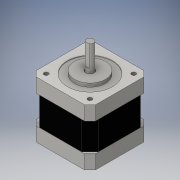
# Autodesk Inventor part: nema17_40mm
Saved by Autodesk Inventor 2016 (Build 200138000, 138)
## iProperties
Created: 2016-06-20
Part Number: nema17_40mm
Material: Generic
Document SubType Name: Modeling
Designer: brent
Density: 1 g/cm^3
Appearance: Aluminum - Dark
Author: brent
Autodesk Inventor part; units mm, degrees
ref_plane "YZ Plane" through (0, 0, 0) normal (1, 0, 0) x (0, 1, 0)
ref_plane "XZ Plane" through (0, 0, 0) normal (0, 1, 0) x (-1, 0, 0)
sketch "Sketch1" plane through (0, 0, 0) normal (0, 1, 0) x (-1, 0, 0)
  line L0 (-21, 21) -> (21, 21)
  line L1 (21, 21) -> (21, -21)
  line L2 (21, -21) -> (-21, -21)
  line L3 (-21, -21) -> (-21, 21)
  line L4 (-21, 21) -> (21, -21) construction
  line L5 (21, 21) -> (-21, -21) construction
  point P0 (0, 0)
  dimension "d0" = 42
  dimension "d1" = 42
  constraints: 12 end point, 2 midpoint, 2 parallel, 1 horizontal, 1 perpendicular
  measures "d0" distance of L1.end L2.end
  measures "d1" distance of L0.end L1.end
extrude "Extrusion1" add sketch "Sketch1" along normal blind 40
ref_plane "Work Plane1" through (0, 20, 0) normal (0, 1, 0) x (1, 0, 0)
sketch "Sketch2" plane through (0, 40, 0) normal (0, 1, 0) x (1, 0, 0)
  line L0 (0, -38.0423) -> (-38.0423, 0)
  line L1 (-38.0423, 0) -> (0, 38.0423)
  line L2 (0, 38.0423) -> (38.0423, 0)
  line L3 (38.0423, 0) -> (0, -38.0423)
  line L4 (0, -38.0423) -> (0, 38.0423) construction
  line L5 (-38.0423, 0) -> (38.0423, 0) construction
  line L6 (-21, 21) -> (-21, -21) projected
  circle A0 centre (0, 0) radius 250
  dimension "d4" = 53.8
  dimension "d5" = 53.8
  dimension "d6" = 500
  constraints: 12 end point, 2 midpoint, 2 parallel, 2 perpendicular, 1 centre point, 1 coincident
  measures "d4" distance of L0.end L1.end
  measures "d5" distance of L1.end L2.end
  measures "d6" diameter of A0
extrude "Extrusion2" cut sketch "Sketch2" against normal blind 10
sketch "Sketch3" plane through (0, 20, 0) normal (0, 1, 0) x (1, 0, 0)
  line L0 (-20.9, -20.9) -> (20.9, -20.9)
  line L1 (20.9, -20.9) -> (20.9, 20.9)
  line L2 (20.9, 20.9) -> (-20.9, 20.9)
  line L3 (-20.9, 20.9) -> (-20.9, -20.9)
  line L4 (-21, -21) -> (-21, -17.0423) projected
  line L5 (21, -21) -> (17.0423, -21) projected
  line L6 (21, 21) -> (21, 17.0423) projected
  line L7 (-21, 21) -> (-17.0423, 21) projected
  circle A0 centre (0, 0) radius 200
  dimension "d9" = 0.1
  dimension "d10" = 0.1
  dimension "d11" = 0.1
  dimension "d12" = 0.1
  dimension "d13" = 400
  constraints: 8 end point, 2 parallel, 1 centre point, 1 coincident, 1 horizontal, 1 perpendicular
  measures "d9" distance between parallel lines of L4 L3
  measures "d10" distance between parallel lines of L5 L0
  measures "d11" distance between parallel lines of L6 L1
  measures "d12" distance between parallel lines of L7 L2
  measures "d13" diameter of A0
extrude "Extrusion3" cut sketch "Sketch3" along normal up to surface (10 mm away)
chamfer "Chamfer1" distance 6 angle 45 4 edges at (20.9, 25, 20.9) (20.9, 25, -20.9) (-20.9, 25, 20.9) (-20.9, 25, -20.9)
mirror "Mirror1" about plane through (0, 20, 0) normal (0, 1, 0) of "Extrusion3", "Extrusion2", "Chamfer1"
sketch "Sketch4" plane through (0, 40, 0) normal (0, 1, 0) x (1, 0, 0)
  circle A0 centre (0, 0) radius 11
  dimension "d19" = 22
  constraints: 1 centre point, 1 coincident
  measures "d19" diameter of A0
extrude "Extrusion4" add sketch "Sketch4" along normal blind 2
sketch "Sketch5" plane through (0, 40, 0) normal (0, 1, 0) x (1, 0, 0)
  circle A0 centre (0, 0) radius 11 projected
  line L0 (17.0423, -21) -> (21, -17.0423) projected
  line L1 (21, -17.0423) -> (21, 17.0423) projected
  line L2 (21, 17.0423) -> (17.0423, 21) projected
  line L3 (17.0423, 21) -> (-17.0423, 21) projected
  line L4 (-17.0423, 21) -> (-21, 17.0423) projected
  line L5 (-21, 17.0423) -> (-21, -17.0423) projected
  line L6 (-21, -17.0423) -> (-17.0423, -21) projected
  line L7 (-17.0423, -21) -> (17.0423, -21) projected
  circle A1 centre (0, 0) radius 16
  dimension "d22" = 32
  constraints: 1 centre point, 1 coincident
  measures "d22" diameter of A1
extrude "Extrusion5" cut sketch "Sketch5" against normal blind 0.5 contours A1
sketch "Sketch6" plane through (0, 42, 0) normal (0, 1, 0) x (1, 0, 0)
  circle A0 centre (0, 0) radius 3
  dimension "d25" = 6
  constraints: 1 centre point, 1 coincident
  measures "d25" diameter of A0
extrude "Extrusion6" cut sketch "Sketch6" against normal blind 2
sketch "Sketch8" plane through (0, 40, 0) normal (0, 1, 0) x (1, 0, 0)
  circle A0 centre (0, 0) radius 16 construction
  line L0 (17.0423, -21) -> (21, -17.0423) construction
  line L1 (21, -17.0423) -> (21, 17.0423) construction
  line L2 (21, 17.0423) -> (17.0423, 21) construction
  line L3 (17.0423, 21) -> (-17.0423, 21) construction
  line L4 (-17.0423, 21) -> (-21, 17.0423) construction
  line L5 (-21, 17.0423) -> (-21, -17.0423) construction
  line L6 (-21, -17.0423) -> (-17.0423, -21) construction
  line L7 (-17.0423, -21) -> (17.0423, -21) construction
  line L8 (-15.5, -15.5) -> (15.5, -15.5) construction
  line L9 (15.5, -15.5) -> (15.5, 15.5) construction
  line L10 (15.5, 15.5) -> (-15.5, 15.5) construction
  line L11 (-15.5, 15.5) -> (-15.5, -15.5) construction
  line L12 (-15.5, -15.5) -> (15.5, 15.5) construction
  line L13 (15.5, -15.5) -> (-15.5, 15.5) construction
  circle A1 centre (-15.5, 15.5) radius 1.5
  circle A2 centre (15.5, 15.5) radius 1.5
  circle A3 centre (15.5, -15.5) radius 1.5
  circle A4 centre (-15.5, -15.5) radius 1.5
  dimension "d36" = 31
  dimension "d37" = 31
  dimension "d38" = 3
  dimension "d39" = 3
  dimension "d40" = 3
  dimension "d41" = 3
  constraints: 12 end point, 4 centre point, 4 coincident, 2 midpoint, 2 parallel, 1 horizontal, 1 perpendicular
  measures "d36" distance of L10.end L9.end
  measures "d37" distance of L9.end L8.end
  measures "d38" diameter of A1
  measures "d39" diameter of A2
  measures "d40" diameter of A3
  measures "d41" diameter of A4
extrude "Extrusion8" cut sketch "Sketch8" against normal blind 5
thread "Thread2" size "M3x0.5" class "6H" standard "ANSI Metric M Profile" full length
sketch "Sketch9" plane through (0, 40, 0) normal (0, 1, 0) x (1, 0, 0)
  circle A0 centre (0, 0) radius 2.5
  dimension "d49" = 5
  constraints: 1 centre point, 1 coincident
  measures "d49" diameter of A0
extrude "Extrusion9" add sketch "Sketch9" along normal blind 20
pattern_circular "Circular Pattern2" count 4 over 360 about axis through (0, 40, 0) along (0, 1, 0) of "Extrusion8"
sketch "Sketch10" plane through (0, 60, 0) normal (0, 1, 0) x (1, 0, 0)
  circle A0 centre (0, 0) radius 2.5 projected
  circle A1 centre (0, 0) radius 2.5 projected
  line L0 (-1.5, -2) -> (1.5, -2)
  line L1 (1.5, -2) -> (1.5, -2.5)
  line L2 (1.5, -2.5) -> (-1.5, -2.5)
  line L3 (-1.5, -2.5) -> (-1.5, -2)
  circle A2 centre (0, 0) radius 2.5 projected
  dimension "d55" = 0.5
  constraints: 8 end point, 2 parallel, 2 point on circle, 1 horizontal, 1 perpendicular, 1 tangent, 2 other
  measures "d55" distance of L0.end L1.end
extrude "Extrusion10" cut sketch "Sketch10" against normal blind 15 contours L0 A0 | A0 L2 L3 | L1 L2 A0 picked at (0.3466, -2.0912)
equation "\"d9\" = d10"
equation "\"d11\" = d10"
equation "\"d12\" = d10"
body "Solid1"
